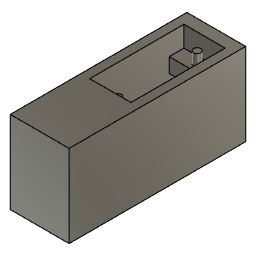
Arm Proto v1 (Autodesk Fusion 360 design; units mm, degrees)
Autodesk Fusion 360 part; units mm, degrees
sketch "Sketch1" plane through (0, 0, 0) normal (0, 0, 1) x (1, 0, 0) in component "Elbow"
  line L0 (10, 30) -> (-10, 30)
  line L1 (-10, 30) -> (-10, -30)
  line L2 (-10, -30) -> (10, -30)
  line L3 (10, -30) -> (10, 30)
  line L4 (10, 30) -> (-10, -30) construction
  line L5 (-10, 30) -> (10, -30) construction
  line L6 (7, 26) -> (-7, 26)
  line L7 (-7, 26) -> (-7, -6)
  line L8 (-7, -6) -> (7, -6)
  line L9 (7, -6) -> (7, 26)
  line L10 (7, 26) -> (-7, -6) construction
  line L11 (-7, 26) -> (7, -6) construction
  point P0 (0, 10)
  constraint perpendicular L0 L1
  constraint parallel L0 L2
  constraint parallel L1 L3
  constraint horizontal L0
  constraint coincident L4 origin
  constraint coincident L5 origin
  constraint perpendicular L6 L7
  constraint parallel L6 L8
  constraint parallel L7 L9
  constraint horizontal L6
  constraint coincident L10 P0
  constraint coincident L11 P0
extrude "Extrude1" add sketch "Sketch1" along normal blind 28 in component "Elbow"
sketch "Sketch2" plane through (0, 0, 0) normal (0, 0, 1) x (1, 0, 0) in component "Elbow"
  line L0 (-7, -6) -> (7, -6)
  line L1 (7, -6) -> (7, -1)
  line L2 (7, -1) -> (-7, -1)
  line L3 (-7, -1) -> (-7, -6)
  line L4 (-7, 26) -> (7, 26)
  line L5 (7, 26) -> (7, 21)
  line L6 (7, 21) -> (-7, 21)
  line L7 (-7, 21) -> (-7, 26)
  constraint horizontal L0
  constraint vertical L1
  constraint horizontal L2
  constraint vertical L3
  constraint horizontal L4
  constraint vertical L5
  constraint horizontal L6
  constraint vertical L7
extrude "Extrude2" add sketch "Sketch2" along normal blind 21 in component "Elbow"
sketch "Sketch3" plane through (0, 0, 0) normal (0, 0, 1) x (1, 0, 0) in component "Elbow"
  line L0 (-7, -1) -> (7, -1)
  line L1 (7, -1) -> (7, -6)
  line L2 (7, -6) -> (-7, -6)
  line L3 (-7, -6) -> (-7, -1)
  line L4 (-7, 26) -> (7, 26)
  line L5 (7, 26) -> (7, 21)
  line L6 (7, 21) -> (-7, 21)
  line L7 (-7, 21) -> (-7, 26)
  constraint horizontal L0
  constraint vertical L1
  constraint horizontal L2
  constraint vertical L3
  constraint horizontal L4
  constraint vertical L5
  constraint horizontal L6
  constraint vertical L7
extrude "Extrude3" cut sketch "Sketch3" along normal blind 16 in component "Elbow"
sketch "Sketch4" plane through (0, 0, 21) normal (0, 0, 1) x (-1, 0, 0) in component "Elbow"
  line L0 (7, 1) -> (7, 6)
  line L1 (7, 6) -> (-7, 6)
  line L2 (-7, 6) -> (-7, 1)
  line L3 (-7, 1) -> (7, 1)
  circle A0 centre (0, 3.5) radius 1.25
  dimension "d7" = 2.5
  measures "d7" diameter of A0
extrude "Extrude4" add sketch "Sketch4" along normal blind 4 contours A0 in component "Elbow"
sketch "Sketch5" plane through (0, 0, 21) normal (0, 0, 1) x (-1, 0, 0) in component "Elbow"
  line L0 (7, -21) -> (-7, -21)
  line L1 (-7, -21) -> (-7, -26)
  line L2 (-7, -26) -> (7, -26)
  line L3 (7, -26) -> (7, -21)
  circle A0 centre (0, -23.5) radius 1.25
  dimension "d10" = 2.5
  measures "d10" diameter of A0
extrude "Extrude5" add sketch "Sketch5" along normal blind 4 contours A0 in component "Elbow"
component "Elbow" placed x (1, 0, 0) y (0, 1, 0) z (0, 0, 1) at (0, 0, 0)
